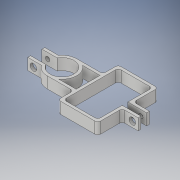
# Autodesk Inventor part: kinect mount
Saved by Autodesk Inventor 2018 (Build 220112000, 112)
## iProperties
Created: 2018-01-11
Part Number: kinect mount
Material: Generic
Document SubType Name: Modeling
Designer: prakh
Density: 1 g/cm^3
Appearance: Default
Author: prakh
Autodesk Inventor part; units mm, degrees
ref_plane "YZ Plane" through (0, 0, 0) normal (1, 0, 0) x (0, 1, 0)
ref_plane "XZ Plane" through (0, 0, 0) normal (0, 1, 0) x (-1, 0, 0)
ref_plane "XY Plane" through (0, 0, 0) normal (0, 0, 1) x (1, 0, 0)
sketch "Sketch1" plane through (0, 0, 0) normal (0, 1, 0) x (-1, 0, 0)
  line L0 (0, 0) -> (38.1, 0)
  line L1 (38.1, 0) -> (38.1, -60.96)
  line L2 (38.1, -60.96) -> (0, -60.96)
  line L3 (-3.175, 3.175) -> (41.275, 3.175)
  line L4 (41.275, 3.175) -> (41.275, -64.135)
  line L5 (41.275, -64.135) -> (-3.175, -64.135)
  line L6 (-3.175, -36.83) -> (-20.955, -36.83)
  line L7 (-20.955, -36.83) -> (-20.955, -33.655)
  line L8 (-20.955, -33.655) -> (0, -33.655)
  line L9 (0, -33.655) -> (0, -44.417)
  line L10 (-3.175, -24.13) -> (-20.955, -24.13)
  line L11 (-20.955, -24.13) -> (-20.955, -27.305)
  line L12 (-20.955, -27.305) -> (0, -27.305)
  line L13 (0, -27.305) -> (0, -17.217)
  line L14 (0, -60.96) -> (0, -33.655)
  line L15 (0, -27.305) -> (0, 0)
  line L16 (-3.175, -24.13) -> (-3.175, 3.175)
  line L17 (-3.175, -64.135) -> (-3.175, -36.83)
  arc A0 (82.211, -24.13) -> (82.211, -36.83) centre (70.485, -30.48) ccw
  line L18 (99.2103, -36.83) -> (82.211, -36.83)
  line L19 (99.2103, -40.005) -> (99.2103, -36.83)
  line L20 (82.211, -24.13) -> (99.2103, -24.13)
  line L21 (99.2103, -24.13) -> (99.2103, -20.955)
  line L22 (99.2103, -20.955) -> (83.9703, -20.955)
  line L23 (83.9703, -40.005) -> (99.2103, -40.005)
  arc A1 (83.9703, -20.955) -> (83.9703, -40.005) centre (70.485, -30.48) ccw
  line L24 (41.275, -13.97) -> (70.485, -13.97)
  line L25 (70.485, -46.99) -> (41.275, -46.99)
  line L26 (60.7506, -17.145) -> (41.275, -17.145)
  line L27 (60.7506, -43.815) -> (41.275, -43.815)
  point P0 (41.275, -30.48)
  dimension "d0" = 38.1
  dimension "d1" = 60.96
  dimension "d2" = 3.175
  dimension "d3" = 3.175
  dimension "d4" = 3.175
  dimension "d5" = 3.175
  dimension "d6" = 3.175
  dimension "d7" = 3.175
  dimension "d8" = 3.175
  dimension "d9" = 17.78
  dimension "d10" = 6.35
  dimension "d23" = 26.67
  dimension "d25" = 3.175
  dimension "d27" = 15.24
  dimension "d28" = 6.35
  dimension "d29" = 6.35
  dimension "d30" = 3.175
  dimension "d31" = 3.175
  dimension "d32" = 12.7
  dimension "d33" = 3.175
  dimension "d34" = 3.175
  constraints: 56 end point, 14 parallel, 8 point on circle, 7 perpendicular, 6 horizontal, 6 point on line, 4 collinear, 2 centre point, 2 tangent, 1 coincident, 1 horizontal alignment, 1 midpoint
  measures "d0" distance of L1.end L2.end
  measures "d1" distance of L0.end L1.end
  measures "d2" distance between parallel lines of L4 L1
  measures "d3" distance between parallel lines of L5 L2
  measures "d4" distance between parallel lines of L0 L3
  measures "d5" distance between parallel lines of L17 L14
  measures "d6" distance between parallel lines of L15 L16
  measures "d7" distance between parallel lines of L10 L12
  measures "d8" distance between parallel lines of L6 L8
  measures "d9" distance of L10.start L10.end
  measures "d10" distance between parallel lines of L8 L12
  measures "d23" diameter of A0
  measures "d25" distance between parallel lines of L22 L20
  measures "d27" distance of L23.start L19.start
  measures "d28" distance from line of A0.centre L18
  measures "d29" distance from line of A0.centre L20
  measures "d30" distance between parallel lines of L23 L18
  measures "d31" radial gap between concentric circles of A0 A1
  measures "d32" distance edge to line of A1 L4
  measures "d33" distance between parallel lines of L25 L27
  measures "d34" distance between parallel lines of L24 L26
extrude "Extrusion1" add sketch "Sketch1" along normal blind 12.7 contours L15 L13 L12 L11 L10 L16 L3 L4 L5 L17 L6 L7 L8 L9 L14 L2 L1 L0 | L24 A1 L26 L4 | A1 L22 L21 L20 A0 L18 L19 L23 | L27 A1 L25 L4
sketch "Sketch2" plane through (3.175, 0, -24.13) normal (0, 0, 1) x (1, 0, 0)
  circle A0 centre (11.43, 6.35) radius 2.4638
  line L0 (0, 12.7) -> (17.78, 12.7) projected
  line L1 (17.78, 0) -> (17.78, 12.7) projected
  point P0 (-3.175, 0)
  dimension "d13" = 4.9276
  dimension "d14" = 6.35
  dimension "d15" = 6.35
  constraints: 1 centre point
  measures "d13" diameter of A0
  measures "d14" distance from line of A0.centre L0
  measures "d15" distance from line of A0.centre L1
extrude "Extrusion2" cut sketch "Sketch2" against normal blind 23.8125
sketch "Sketch3" plane through (3.175, 0, -24.13) normal (0, 0, 1) x (1, 0, 0)
  circle A0 centre (11.43, 6.35) radius 2.4638 projected
  circle A1 centre (11.43, 6.35) radius 3.7338
  point P0 (-3.175, 0)
  dimension "d18" = 1.27
  constraints: 1 centre point, 1 coincident
  measures "d18" radial gap between concentric circles of A0 A1
extrude "Extrusion3" cut sketch "Sketch3" against normal blind 9.525
fillet "Fillet1" radius 3.175 4 edges at (-38.1, 6.35, -60.96) (0, 6.35, -60.96) (0, 6.35, 0) (-38.1, 6.35, 0)
fillet "Fillet2" radius 3.175 8 edges at (-41.275, 6.35, 3.175) (-41.275, 6.35, -64.135) (3.175, 6.35, -64.135) (3.175, 6.35, 3.175) (3.175, 6.35, -24.13) (3.175, 6.35, -36.83) (-41.275, 6.35, -13.97) (-41.275, 6.35, -46.99)
sketch "Sketch4" plane through (-99.2103, 0, -20.955) normal (0, 0, 1) x (1, 0, 0)
  circle A0 centre (6.35, 6.35) radius 2.4638
  line L0 (0, 12.7) -> (15.24, 12.7) projected
  line L1 (0, 0) -> (0, 12.7) projected
  point P0 (99.2103, 0)
  dimension "d35" = 4.9276
  dimension "d36" = 6.35
  dimension "d37" = 6.35
  constraints: 1 centre point
  measures "d35" diameter of A0
  measures "d36" distance from line of A0.centre L0
  measures "d37" distance from line of A0.centre L1
extrude "Extrusion4" cut sketch "Sketch4" against normal blind 23.8125
sketch "Sketch5" plane through (-99.2103, 0, -20.955) normal (0, 0, 1) x (1, 0, 0)
  circle A0 centre (6.35, 6.35) radius 2.4638 projected
  circle A1 centre (6.35, 6.35) radius 3.7338
  point P0 (99.2103, 0)
  dimension "d40" = 1.27
  constraints: 1 centre point, 1 coincident
  measures "d40" radial gap between concentric circles of A1 A0
extrude "Extrusion5" cut sketch "Sketch5" against normal blind 9.525
equation "\"d3\" = d2"
equation "\"d4\" = d2"
equation "\"d5\" = d2"
equation "\"d6\" = d2"
equation "\"d7\" = d2"
equation "\"d8\" = d2"
equation "\"d25\" = d2"
equation "\"d29\" = d28"
equation "\"d30\" = d2"
equation "\"d31\" = d2"
equation "\"d33\" = d2"
equation "\"d34\" = d2"
equation "\"d15\" = d14"
equation "\"d37\" = d36"
equation "\"d24\" = d2"
equation "\"d26\" = d2"
body "Solid1"
